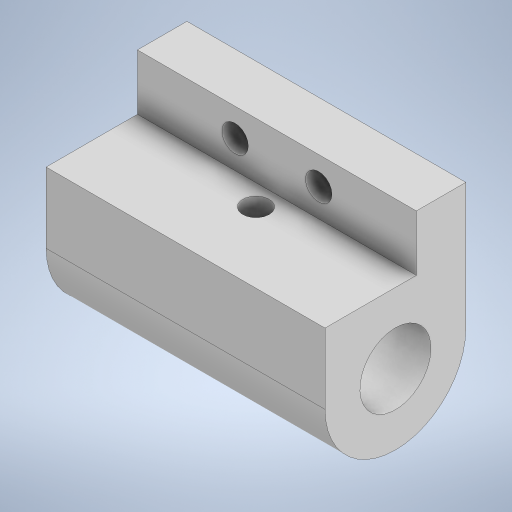
# Autodesk Inventor part: arm_to_camera
Saved by Autodesk Inventor 2024 (Build 280153000, 153)
## iProperties
Created: 2023-10-26
Part Number: arm_to_camera
Material: Generic
Document SubType Name: Modeling
Designer: dimademler
Density: 1 g/cm^3
Appearance: Default
Author: dimademler
Autodesk Inventor part; units mm, degrees
ref_plane "YZ Plane" through (0, 0, 0) normal (1, 0, 0) x (0, 1, 0)
ref_plane "XZ Plane" through (0, 0, 0) normal (0, 1, 0) x (-1, 0, 0)
ref_plane "XY Plane" through (0, 0, 0) normal (0, 0, 1) x (1, 0, 0)
sketch "Sketch1" plane through (0, 0, 0) normal (1, 0, 0) x (0, 1, 0)
  circle A0 centre (0, 0) radius 6.477
  circle A1 centre (0, 0) radius 12.827
  dimension "d0" = 12.954
  dimension "d1" = 25.654
  constraints: 2 centre point, 2 coincident
  measures "d0" diameter of A0
  measures "d1" diameter of A1
extrude "Extrusion1" add sketch "Sketch1" along normal blind 50.8
sketch "Sketch2" plane through (50.8, 0, 0) normal (1, 0, 0) x (0, 0, -1)
  circle A0 centre (0, 0) radius 12.827 projected
  circle A1 centre (0, 0) radius 6.477 projected
  line L0 (0, 0) -> (0, 12.827) construction
  line L1 (0, 12.827) -> (-3.81, 12.827)
  arc A2 (-12.827, 0) -> (12.827, 0) centre (0, 0) ccw construction
  line L2 (0, 0) -> (12.827, 0) construction
  line L3 (0, 0) -> (-12.827, 0) construction
  line L4 (-12.827, 0) -> (-12.827, 12.827)
  line L5 (-12.827, 12.827) -> (0, 12.827)
  line L6 (12.827, 12.827) -> (12.827, 0)
  circle A3 centre (0, 0) radius 12.827 projected
  line L7 (12.827, 12.827) -> (3.81, 12.827) construction
  arc A4 (0, 12.827) -> (-12.827, 0) centre (0, 0) ccw
  arc A5 (12.827, 0) -> (0, 12.827) centre (0, 0) ccw
  line L8 (0, 12.827) -> (3.81, 12.827)
  line L9 (3.81, 12.827) -> (3.81, 22.987)
  line L10 (3.81, 22.987) -> (12.827, 22.987)
  line L11 (12.827, 22.987) -> (12.827, 12.827)
  line L12 (3.81, 12.827) -> (0, 12.827)
  point P0 (12.827, 0)
  dimension "d5" = 3.81
  dimension "d6" = 10.16
  constraints: 26 end point, 13 tangent, 6 point on circle, 5 horizontal, 5 perpendicular, 3 centre point, 3 vertical, 2 point on line, 1 coincident, 3 other
  measures "d5" distance of L0.end L7.end
  measures "d6" distance of L7.end L9.end
extrude "Extrusion2" add sketch "Sketch2" against normal blind 50.8 contours A0 L8 L9 L10 L11 L6 | A0 L4 L5 L1
sketch "Sketch3" plane through (50.8, 12.827, -3.81) normal (0, 0, 1) x (1, 0, 0)
  line L0 (0, 0) -> (-50.8, 0) projected
  line L1 (0, 10.16) -> (-50.8, 10.16) projected
  line L2 (-50.8, 0) -> (-50.8, 10.16) projected
  line L3 (0, 10.16) -> (0, 0) projected
  line L4 (-25.4, 10.16) -> (-25.4, 0) construction
  line L5 (-25.4, 5.08) -> (-17.78, 5.08) construction
  circle A0 centre (-17.78, 5.08) radius 2.413
  circle A1 centre (-33.02, 5.08) radius 2.413
  point P0 (-50.8, -12.827)
  dimension "d9" = 7.62
  dimension "d11" = 4.826
  constraints: 4 end point, 3 midpoint, 2 centre point, 1 coincident, 1 horizontal, 1 symmetric about line, 1 other
  measures "d9" distance of L5.start L5.end
  measures "d11" diameter of A0
extrude "Extrusion3" cut sketch "Sketch3" against normal through all contours A0 | A1
sketch "Sketch4" plane through (50.8, 12.827, 12.827) normal (0, 1, 0) x (1, 0, 0)
  line L0 (0, 16.637) -> (0, 0) projected
  line L1 (0, 16.637) -> (-50.8, 16.637) projected
  line L2 (-50.8, 0) -> (-50.8, 16.637) projected
  line L3 (0, 0) -> (-50.8, 0) projected
  line L4 (-25.4, 0) -> (-25.4, 16.637) construction
  line L5 (0, 19.304) -> (0, 6.35) projected
  line L6 (0, 12.827) -> (-50.8, 12.827) construction
  circle A0 centre (-25.4, 12.827) radius 2.413
  dimension "d15" = 4.826
  constraints: 4 end point, 4 midpoint, 1 centre point, 1 horizontal
  measures "d15" diameter of A0
extrude "Extrusion4" cut sketch "Sketch4" against normal through all contours A0
body "Solid1"
